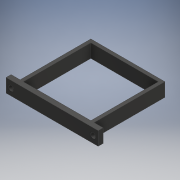
# Autodesk Inventor part: soporteMatrizInferior
Saved by Autodesk Inventor 2017 (Build 210142000, 142)
## iProperties
Part Number: soporteMatrizInferior
Material: Genérico
Document SubType Name: Modeling
Designer: Roberto
Density: 1 g/cm^3
Appearance: Valor por defecto
Author: Roberto
Autodesk Inventor part; units mm, degrees
ref_plane "YZ Plane" through (0, 0, 0) normal (1, 0, 0) x (0, 1, 0)
ref_plane "XZ Plane" through (0, 0, 0) normal (0, 1, 0) x (-1, 0, 0)
ref_plane "XY Plane" through (0, 0, 0) normal (0, 0, 1) x (1, 0, 0)
sketch "Boceto1" plane through (0, 0, 0) normal (0, 1, 0) x (-1, 0, 0)
  circle A0 centre (-5.172, -0.4) radius 0.15
  circle A1 centre (-0.3, -0.4) radius 0.15
  line L0 (-5.472, 0) -> (-5.472, -0.8)
  line L1 (0, 0) -> (0, -0.8)
  line L2 (0, 0) -> (-5.472, 0)
  line L3 (-4.736, -0.8) -> (-4.936, -0.8)
  line L4 (-4.736, 0) -> (-4.936, 0)
  line L5 (-4.936, -0.8) -> (-4.936, -1)
  line L6 (-4.936, -1) -> (-0.536, -1)
  line L7 (-0.536, -1) -> (-0.536, -0.8)
  line L8 (0, -0.8) -> (-0.536, -0.8)
  line L9 (-4.936, -0.8) -> (-5.472, -0.8)
  dimension "d1" = 1
  constraints: 20 end point, 3 perpendicular, 2 centre point, 2 point on line
  measures "d1" distance of L4.end L5.end
extrude "Extrusión1" add sketch "Boceto1" along normal blind 0.3
sketch "Boceto2" plane through (0, 0.3, 0) normal (0, 1, 0) x (1, 0, 0)
  line L0 (4.936, 1) -> (0.536, 1) projected
  line L1 (0.536, 1) -> (0.536, 0)
  line L2 (0.536, 0) -> (0.736, 0)
  line L3 (0.736, 0) -> (0.736, 0.8)
  line L4 (0.736, 0.8) -> (4.736, 0.8)
  line L5 (4.736, 0.8) -> (4.736, 0)
  line L6 (4.736, 0) -> (4.936, 0)
  line L7 (4.936, 0) -> (4.936, 1)
  line L8 (0.536, 1) -> (0.536, 0.8) projected
  line L9 (4.936, 1) -> (0.536, 1)
  dimension "d5" = 0.2
  dimension "d6" = 4
  constraints: 16 end point, 4 perpendicular, 2 point on line, 1 horizontal, 1 vertical
  measures "d5" distance of L1.end L2.end
  measures "d6" distance of L3.end L4.end
extrude "Extrusión2" add sketch "Boceto2" along normal blind 4
sketch "Boceto3" plane through (0, 4.3, 0) normal (0, 1, 0) x (1, 0, 0)
  line L0 (0.536, 1) -> (0.536, 0) projected
  line L1 (4.936, 1) -> (0.536, 1) projected
  line L2 (0.536, 0) -> (4.936, 0)
  line L3 (4.936, 0) -> (4.936, 1)
  line L4 (4.936, 1) -> (0.536, 1)
  line L5 (0.536, 1) -> (0.536, 0)
  point P0 (0, 0)
  constraints: 8 end point, 2 parallel, 1 horizontal, 1 perpendicular
extrude "Extrusión3" add sketch "Boceto3" along normal blind 0.2
sketch "Boceto5" plane through (0, 0, 0) normal (0, -1, 0) x (1, 0, 0)
  circle A0 centre (0.3, -0.4) radius 0.15 projected
  circle A1 centre (5.172, -0.4) radius 0.15 projected
  line L0 (5.472, 0) -> (5.472, -0.8) projected
  line L1 (0, 0) -> (5.472, 0) projected
  line L2 (0, -0.8) -> (0, 0) projected
  line L3 (0.536, -0.8) -> (0, -0.8) projected
  line L4 (0.536, -1) -> (0.536, -0.8) projected
  line L5 (4.936, -1) -> (0.536, -1) projected
  line L6 (4.936, -0.8) -> (4.936, -1) projected
  line L7 (5.472, -0.8) -> (4.936, -0.8) projected
  line L8 (4.936, -0.8) -> (0.536, -0.8)
  line L9 (0.536, -0.8) -> (0.536, -1)
  line L10 (0.536, -1) -> (4.936, -1)
  line L11 (4.936, -1) -> (4.936, -0.8)
  constraints: 8 end point, 2 parallel, 1 horizontal, 1 perpendicular
extrude "Extrusión5" cut sketch "Boceto5" against normal blind 20 contours L6 L5 L4 L8
